Autodesk Inventor part; units mm, degrees
(part 6 of 6)
  line L4697 (26, 19.883) -> (26, 20.883)
  line L4698 (26, 20.883) -> (25, 20.883)
  line L4699 (25, 20.883) -> (25, 19.883)
  line L4700 (25, 20.383) -> (26, 20.383)
  line L4701 (26, 20.383) -> (26, 21.383)
  line L4702 (26, 21.383) -> (25, 21.383)
  line L4703 (25, 21.383) -> (25, 20.383)
  line L4704 (25, 20.883) -> (26, 20.883)
  line L4705 (26, 20.883) -> (26, 21.883)
  line L4706 (26, 21.883) -> (25, 21.883)
  line L4707 (25, 21.883) -> (25, 20.883)
  line L4708 (25, 21.383) -> (26, 21.383)
  line L4709 (26, 21.383) -> (26, 22.383)
  line L4710 (26, 22.383) -> (25, 22.383)
  line L4711 (25, 22.383) -> (25, 21.383)
  line L4712 (25, 21.883) -> (26, 21.883)
  line L4713 (26, 21.883) -> (26, 22.883)
  line L4714 (26, 22.883) -> (25, 22.883)
  line L4715 (25, 22.883) -> (25, 21.883)
  line L4716 (23.28, 23.603) -> (24.28, 23.603)
  line L4717 (24.28, 23.603) -> (24.28, 24.603)
  line L4718 (24.28, 24.603) -> (23.28, 24.603)
  line L4719 (23.28, 24.603) -> (23.28, 23.603)
  line L4720 (22.78, 23.603) -> (23.78, 23.603)
  line L4721 (23.78, 23.603) -> (23.78, 24.603)
  line L4722 (23.78, 24.603) -> (22.78, 24.603)
  line L4723 (22.78, 24.603) -> (22.78, 23.603)
  line L4724 (22.28, 23.603) -> (23.28, 23.603)
  line L4725 (23.28, 23.603) -> (23.28, 24.603)
  line L4726 (23.28, 24.603) -> (22.28, 24.603)
  line L4727 (22.28, 24.603) -> (22.28, 23.603)
  line L4728 (21.78, 23.603) -> (22.78, 23.603)
  line L4729 (22.78, 23.603) -> (22.78, 24.603)
  line L4730 (22.78, 24.603) -> (21.78, 24.603)
  line L4731 (21.78, 24.603) -> (21.78, 23.603)
  line L4732 (21.28, 23.603) -> (22.28, 23.603)
  line L4733 (22.28, 23.603) -> (22.28, 24.603)
  line L4734 (22.28, 24.603) -> (21.28, 24.603)
  line L4735 (21.28, 24.603) -> (21.28, 23.603)
  line L4736 (20.78, 23.603) -> (21.78, 23.603)
  line L4737 (21.78, 23.603) -> (21.78, 24.603)
  line L4738 (21.78, 24.603) -> (20.78, 24.603)
  line L4739 (20.78, 24.603) -> (20.78, 23.603)
  line L4740 (20.28, 23.603) -> (21.28, 23.603)
  line L4741 (21.28, 23.603) -> (21.28, 24.603)
  line L4742 (21.28, 24.603) -> (20.28, 24.603)
  line L4743 (20.28, 24.603) -> (20.28, 23.603)
  line L4744 (19.78, 23.603) -> (20.78, 23.603)
  line L4745 (20.78, 23.603) -> (20.78, 24.603)
  line L4746 (20.78, 24.603) -> (19.78, 24.603)
  line L4747 (19.78, 24.603) -> (19.78, 23.603)
  line L4748 (19.28, 23.603) -> (20.28, 23.603)
  line L4749 (20.28, 23.603) -> (20.28, 24.603)
  line L4750 (20.28, 24.603) -> (19.28, 24.603)
  line L4751 (19.28, 24.603) -> (19.28, 23.603)
  line L4752 (18.78, 23.603) -> (19.78, 23.603)
  line L4753 (19.78, 23.603) -> (19.78, 24.603)
  line L4754 (19.78, 24.603) -> (18.78, 24.603)
  line L4755 (18.78, 24.603) -> (18.78, 23.603)
  line L4756 (18.28, 23.603) -> (19.28, 23.603)
  line L4757 (19.28, 23.603) -> (19.28, 24.603)
  line L4758 (19.28, 24.603) -> (18.28, 24.603)
  line L4759 (18.28, 24.603) -> (18.28, 23.603)
  line L4760 (17.78, 23.603) -> (18.78, 23.603)
  line L4761 (18.78, 23.603) -> (18.78, 24.603)
  line L4762 (18.78, 24.603) -> (17.78, 24.603)
  line L4763 (17.78, 24.603) -> (17.78, 23.603)
  line L4764 (17.28, 23.603) -> (18.28, 23.603)
  line L4765 (18.28, 23.603) -> (18.28, 24.603)
  line L4766 (18.28, 24.603) -> (17.28, 24.603)
  line L4767 (17.28, 24.603) -> (17.28, 23.603)
  line L4768 (16.78, 23.603) -> (17.78, 23.603)
  line L4769 (17.78, 23.603) -> (17.78, 24.603)
  line L4770 (17.78, 24.603) -> (16.78, 24.603)
  line L4771 (16.78, 24.603) -> (16.78, 23.603)
  line L4772 (16.28, 23.603) -> (17.28, 23.603)
  line L4773 (17.28, 23.603) -> (17.28, 24.603)
  line L4774 (17.28, 24.603) -> (16.28, 24.603)
  line L4775 (16.28, 24.603) -> (16.28, 23.603)
  line L4776 (15.78, 23.603) -> (16.78, 23.603)
  line L4777 (16.78, 23.603) -> (16.78, 24.603)
  line L4778 (16.78, 24.603) -> (15.78, 24.603)
  line L4779 (15.78, 24.603) -> (15.78, 23.603)
  line L4780 (15.28, 23.603) -> (16.28, 23.603)
  line L4781 (16.28, 23.603) -> (16.28, 24.603)
  line L4782 (16.28, 24.603) -> (15.28, 24.603)
  line L4783 (15.28, 24.603) -> (15.28, 23.603)
  line L4784 (14.78, 23.603) -> (15.78, 23.603)
  line L4785 (15.78, 23.603) -> (15.78, 24.603)
  line L4786 (15.78, 24.603) -> (14.78, 24.603)
  line L4787 (14.78, 24.603) -> (14.78, 23.603)
  line L4788 (14.28, 23.603) -> (15.28, 23.603)
  line L4789 (15.28, 23.603) -> (15.28, 24.603)
  line L4790 (15.28, 24.603) -> (14.28, 24.603)
  line L4791 (14.28, 24.603) -> (14.28, 23.603)
  line L4792 (13.78, 23.603) -> (14.78, 23.603)
  line L4793 (14.78, 23.603) -> (14.78, 24.603)
  line L4794 (14.78, 24.603) -> (13.78, 24.603)
  line L4795 (13.78, 24.603) -> (13.78, 23.603)
  line L4796 (13.28, 23.603) -> (14.28, 23.603)
  line L4797 (14.28, 23.603) -> (14.28, 24.603)
  line L4798 (14.28, 24.603) -> (13.28, 24.603)
  line L4799 (13.28, 24.603) -> (13.28, 23.603)
  line L4800 (12.78, 23.603) -> (13.78, 23.603)
  line L4801 (13.78, 23.603) -> (13.78, 24.603)
  line L4802 (13.78, 24.603) -> (12.78, 24.603)
  line L4803 (12.78, 24.603) -> (12.78, 23.603)
  line L4804 (12.28, 23.603) -> (13.28, 23.603)
  line L4805 (13.28, 23.603) -> (13.28, 24.603)
  line L4806 (13.28, 24.603) -> (12.28, 24.603)
  line L4807 (12.28, 24.603) -> (12.28, 23.603)
  line L4808 (11.78, 23.603) -> (12.78, 23.603)
  line L4809 (12.78, 23.603) -> (12.78, 24.603)
  line L4810 (12.78, 24.603) -> (11.78, 24.603)
  line L4811 (11.78, 24.603) -> (11.78, 23.603)
  line L4812 (11.28, 23.603) -> (12.28, 23.603)
  line L4813 (12.28, 23.603) -> (12.28, 24.603)
  line L4814 (12.28, 24.603) -> (11.28, 24.603)
  line L4815 (11.28, 24.603) -> (11.28, 23.603)
  circle A74 centre (19.9, 34.55) radius 0.17
  circle A75 centre (19.1, 34.55) radius 0.17
  circle A76 centre (18.3, 34.55) radius 0.17
  circle A77 centre (17.5, 34.55) radius 0.17
  circle A78 centre (16.7, 34.55) radius 0.17
  circle A79 centre (15.9, 34.55) radius 0.17
  circle A80 centre (19.9, 35.3) radius 0.17
  circle A81 centre (19.1, 35.3) radius 0.17
  circle A82 centre (18.3, 35.3) radius 0.17
  circle A83 centre (17.5, 35.3) radius 0.17
  circle A84 centre (16.7, 35.3) radius 0.17
  circle A85 centre (15.9, 35.3) radius 0.17
  circle A86 centre (19.9, 36.05) radius 0.17
  circle A87 centre (15.9, 36.05) radius 0.17
  circle A88 centre (19.9, 36.8) radius 0.17
  circle A89 centre (15.9, 36.8) radius 0.17
  circle A90 centre (19.9, 37.55) radius 0.17
  circle A91 centre (19.1, 37.55) radius 0.17
  circle A92 centre (18.3, 37.55) radius 0.17
  circle A93 centre (17.5, 37.55) radius 0.17
  circle A94 centre (16.7, 37.55) radius 0.17
  circle A95 centre (15.9, 37.55) radius 0.17
  circle A96 centre (19.9, 38.3) radius 0.17
  circle A97 centre (19.1, 38.3) radius 0.17
  circle A98 centre (18.3, 38.3) radius 0.17
  circle A99 centre (17.5, 38.3) radius 0.17
  circle A100 centre (16.7, 38.3) radius 0.17
  circle A101 centre (15.9, 38.3) radius 0.17
  line L4816 (8.103, 5.199) -> (8.103, 4.199)
  line L4817 (8.103, 4.199) -> (9.103, 4.199)
  line L4818 (9.103, 4.199) -> (9.103, 5.199)
  line L4819 (9.103, 5.199) -> (8.103, 5.199)
  line L4820 (8.103, 3.929) -> (8.103, 2.929)
  line L4821 (8.103, 2.929) -> (9.103, 2.929)
  line L4822 (9.103, 2.929) -> (9.103, 3.929)
  line L4823 (9.103, 3.929) -> (8.103, 3.929)
  line L4824 (8.103, 2.659) -> (8.103, 1.659)
  line L4825 (8.103, 1.659) -> (9.103, 1.659)
  line L4826 (9.103, 1.659) -> (9.103, 2.659)
  line L4827 (9.103, 2.659) -> (8.103, 2.659)
  line L4828 (8.103, 1.389) -> (8.103, 0.389)
  line L4829 (8.103, 0.389) -> (9.103, 0.389)
  line L4830 (9.103, 0.389) -> (9.103, 1.389)
  line L4831 (9.103, 1.389) -> (8.103, 1.389)
  line L4832 (13.503, 1.389) -> (13.503, 0.389)
  line L4833 (13.503, 0.389) -> (14.503, 0.389)
  line L4834 (14.503, 0.389) -> (14.503, 1.389)
  line L4835 (14.503, 1.389) -> (13.503, 1.389)
  line L4836 (13.503, 2.659) -> (13.503, 1.659)
  line L4837 (13.503, 1.659) -> (14.503, 1.659)
  line L4838 (14.503, 1.659) -> (14.503, 2.659)
  line L4839 (14.503, 2.659) -> (13.503, 2.659)
  line L4840 (13.503, 3.929) -> (13.503, 2.929)
  line L4841 (13.503, 2.929) -> (14.503, 2.929)
  line L4842 (14.503, 2.929) -> (14.503, 3.929)
  line L4843 (14.503, 3.929) -> (13.503, 3.929)
  line L4844 (13.503, 5.199) -> (13.503, 4.199)
  line L4845 (13.503, 4.199) -> (14.503, 4.199)
  line L4846 (14.503, 4.199) -> (14.503, 5.199)
  line L4847 (14.503, 5.199) -> (13.503, 5.199)
  line L4848 (10.803, 3.294) -> (10.803, 2.294)
  line L4849 (10.803, 2.294) -> (11.803, 2.294)
  line L4850 (11.803, 2.294) -> (11.803, 3.294)
  line L4851 (11.803, 3.294) -> (10.803, 3.294)
  line L4852 (31.641, 22.218) -> (31.641, 21.068)
  line L4853 (31.641, 21.068) -> (32.791, 21.068)
  line L4854 (32.791, 21.068) -> (32.791, 22.218)
  line L4855 (32.791, 22.218) -> (31.641, 22.218)
  line L4856 (34.266, 22.143) -> (34.266, 21.143)
  line L4857 (34.266, 21.143) -> (35.266, 21.143)
  line L4858 (35.266, 21.143) -> (35.266, 22.143)
  line L4859 (35.266, 22.143) -> (34.266, 22.143)
  line L4860 (32.166, 32.593) -> (32.166, 31.593)
  line L4861 (32.166, 31.593) -> (33.166, 31.593)
  line L4862 (33.166, 31.593) -> (33.166, 32.593)
  line L4863 (33.166, 32.593) -> (32.166, 32.593)
  line L4864 (33.366, 32.793) -> (33.366, 31.793)
  line L4865 (33.366, 31.793) -> (34.366, 31.793)
  line L4866 (34.366, 31.793) -> (34.366, 32.793)
  line L4867 (34.366, 32.793) -> (33.366, 32.793)
  line L4868 (34.416, 32.593) -> (34.416, 31.593)
  line L4869 (34.416, 31.593) -> (35.416, 31.593)
  line L4870 (35.416, 31.593) -> (35.416, 32.593)
  line L4871 (35.416, 32.593) -> (34.416, 32.593)
  line L4872 (30.666, 30.943) -> (30.666, 29.943)
  line L4873 (30.666, 29.943) -> (31.666, 29.943)
  line L4874 (31.666, 29.943) -> (31.666, 30.943)
  line L4875 (31.666, 30.943) -> (30.666, 30.943)
  line L4876 (30.666, 29.843) -> (30.666, 28.843)
  line L4877 (30.666, 28.843) -> (31.666, 28.843)
  line L4878 (31.666, 28.843) -> (31.666, 29.843)
  line L4879 (31.666, 29.843) -> (30.666, 29.843)
  line L4880 (30.666, 28.743) -> (30.666, 27.743)
  line L4881 (30.666, 27.743) -> (31.666, 27.743)
  line L4882 (31.666, 27.743) -> (31.666, 28.743)
  line L4883 (31.666, 28.743) -> (30.666, 28.743)
  line L4884 (30.666, 27.643) -> (30.666, 26.643)
  line L4885 (30.666, 26.643) -> (31.666, 26.643)
  line L4886 (31.666, 26.643) -> (31.666, 27.643)
  line L4887 (31.666, 27.643) -> (30.666, 27.643)
  line L4888 (30.666, 26.543) -> (30.666, 25.543)
  line L4889 (30.666, 25.543) -> (31.666, 25.543)
  line L4890 (31.666, 25.543) -> (31.666, 26.543)
  line L4891 (31.666, 26.543) -> (30.666, 26.543)
  line L4892 (30.666, 25.443) -> (30.666, 24.443)
  line L4893 (30.666, 24.443) -> (31.666, 24.443)
  line L4894 (31.666, 24.443) -> (31.666, 25.443)
  line L4895 (31.666, 25.443) -> (30.666, 25.443)
  line L4896 (30.666, 24.343) -> (30.666, 23.343)
  line L4897 (30.666, 23.343) -> (31.666, 23.343)
  line L4898 (31.666, 23.343) -> (31.666, 24.343)
  line L4899 (31.666, 24.343) -> (30.666, 24.343)
  line L4900 (30.666, 23.243) -> (30.666, 22.243)
  line L4901 (30.666, 22.243) -> (31.666, 22.243)
  line L4902 (31.666, 22.243) -> (31.666, 23.243)
  line L4903 (31.666, 23.243) -> (30.666, 23.243)
  line L4904 (25.87, 4.6275) -> (24.87, 4.6275)
  line L4905 (24.87, 4.6275) -> (24.87, 3.6275)
  line L4906 (24.87, 3.6275) -> (25.87, 3.6275)
  line L4907 (25.87, 3.6275) -> (25.87, 4.6275)
  line L4908 (26.52, 4.6275) -> (25.52, 4.6275)
  line L4909 (25.52, 4.6275) -> (25.52, 3.6275)
  line L4910 (25.52, 3.6275) -> (26.52, 3.6275)
  line L4911 (26.52, 3.6275) -> (26.52, 4.6275)
  line L4912 (27.17, 4.6275) -> (26.17, 4.6275)
  line L4913 (26.17, 4.6275) -> (26.17, 3.6275)
  line L4914 (26.17, 3.6275) -> (27.17, 3.6275)
  line L4915 (27.17, 3.6275) -> (27.17, 4.6275)
  line L4916 (27.82, 4.6275) -> (26.82, 4.6275)
  line L4917 (26.82, 4.6275) -> (26.82, 3.6275)
  line L4918 (26.82, 3.6275) -> (27.82, 3.6275)
  line L4919 (27.82, 3.6275) -> (27.82, 4.6275)
  line L4920 (28.47, 4.6275) -> (27.47, 4.6275)
  line L4921 (27.47, 4.6275) -> (27.47, 3.6275)
  line L4922 (27.47, 3.6275) -> (28.47, 3.6275)
  line L4923 (28.47, 3.6275) -> (28.47, 4.6275)
  circle A102 centre (23.37, 1.4525) radius 0.935
  circle A103 centre (23.37, 1.4525) radius 0.935
  circle A104 centre (23.37, 1.4525) radius 0.935
  circle A105 centre (23.37, 1.4525) radius 0.935
  circle A106 centre (29.97, 1.4525) radius 0.935
  circle A107 centre (29.97, 1.4525) radius 0.935
  circle A108 centre (29.97, 1.4525) radius 0.935
  circle A109 centre (29.97, 1.4525) radius 0.935
  line L4924 (23.97, 3.6275) -> (23.97, 4.6275)
  line L4925 (23.97, 4.6275) -> (22.97, 4.6275)
  line L4926 (22.97, 4.6275) -> (22.97, 3.6275)
  line L4927 (22.97, 3.6275) -> (23.97, 3.6275)
  line L4928 (30.37, 3.6275) -> (30.37, 4.6275)
  line L4929 (30.37, 4.6275) -> (29.37, 4.6275)
  line L4930 (29.37, 4.6275) -> (29.37, 3.6275)
  line L4931 (29.37, 3.6275) -> (30.37, 3.6275)
  line L4932 (24.52, 0.5025) -> (26.42, 0.5025)
  line L4933 (26.42, 0.5025) -> (26.42, 2.4025)
  line L4934 (26.42, 2.4025) -> (24.52, 2.4025)
  line L4935 (24.52, 2.4025) -> (24.52, 0.5025)
  line L4936 (26.92, 0.5025) -> (28.82, 0.5025)
  line L4937 (28.82, 0.5025) -> (28.82, 2.4025)
  line L4938 (28.82, 2.4025) -> (26.92, 2.4025)
  line L4939 (26.92, 2.4025) -> (26.92, 0.5025)
  line L4940 (4.669, 18.214) -> (4.669, 17.214)
  line L4941 (4.669, 17.214) -> (5.669, 17.214)
  line L4942 (5.669, 17.214) -> (5.669, 18.214)
  line L4943 (5.669, 18.214) -> (4.669, 18.214)
  line L4944 (4.669, 16.364) -> (4.669, 15.364)
  line L4945 (4.669, 15.364) -> (5.669, 15.364)
  line L4946 (5.669, 15.364) -> (5.669, 16.364)
  line L4947 (5.669, 16.364) -> (4.669, 16.364)
  line L4948 (6.219, 16.364) -> (6.219, 15.364)
  line L4949 (6.219, 15.364) -> (7.219, 15.364)
  line L4950 (7.219, 15.364) -> (7.219, 16.364)
  line L4951 (7.219, 16.364) -> (6.219, 16.364)
  line L4952 (6.219, 18.214) -> (6.219, 17.214)
  line L4953 (6.219, 17.214) -> (7.219, 17.214)
  line L4954 (7.219, 17.214) -> (7.219, 18.214)
  line L4955 (7.219, 18.214) -> (6.219, 18.214)
  circle A110 centre (29.591, 23.622) radius 0.2286
  circle A111 centre (29.591, 23.622) radius 0.2286
  circle A112 centre (32.385, 14.224) radius 0.2286
  circle A113 centre (32.385, 14.224) radius 0.2286
  circle A114 centre (20.32, 18.034) radius 0.2286
  circle A115 centre (20.32, 18.034) radius 0.2286
  circle A116 centre (13.111, 7.6) radius 0.2286
  circle A117 centre (13.111, 7.6) radius 0.2286
  circle A118 centre (18.7, 37.15) radius 0.2286
  circle A119 centre (18.7, 37.15) radius 0.2286
  circle A120 centre (19.676, 22.67) radius 0.2286
  circle A121 centre (19.676, 22.67) radius 0.2286
  circle A122 centre (16.3, 38.7) radius 0.2286
  circle A123 centre (16.3, 38.7) radius 0.2286
  circle A124 centre (18.149, 21.651) radius 0.2286
  circle A125 centre (18.149, 21.651) radius 0.2286
  circle A126 centre (18.7, 38.7) radius 0.2286
  circle A127 centre (18.7, 38.7) radius 0.2286
  circle A128 centre (20.322, 20.778) radius 0.2286
  circle A129 centre (20.322, 20.778) radius 0.2286
  circle A130 centre (12.78, 35.731) radius 0.2286
  circle A131 centre (12.78, 35.731) radius 0.2286
  circle A132 centre (19.5, 37.15) radius 0.2286
  circle A133 centre (19.5, 37.15) radius 0.2286
  circle A134 centre (13, 22.3) radius 0.2286
  circle A135 centre (13, 22.3) radius 0.2286
  circle A136 centre (13.35, 35) radius 0.2286
  circle A137 centre (13.35, 35) radius 0.2286
  circle A138 centre (20.4, 37.15) radius 0.2286
  circle A139 centre (20.4, 37.15) radius 0.2286
  circle A140 centre (18.9, 28.573) radius 0.2286
  circle A141 centre (18.9, 28.573) radius 0.2286
  circle A142 centre (15.5, 38.7) radius 0.2286
  circle A143 centre (15.5, 38.7) radius 0.2286
  circle A144 centre (14.5, 22.3) radius 0.2286
  circle A145 centre (14.5, 22.3) radius 0.2286
  circle A146 centre (19.5, 38.7) radius 0.2286
  circle A147 centre (19.5, 38.7) radius 0.2286
  circle A148 centre (13.9, 20.7) radius 0.2286
  circle A149 centre (13.9, 20.7) radius 0.2286
  circle A150 centre (15.5, 34.925) radius 0.2286
  circle A151 centre (15.5, 34.925) radius 0.2286
  circle A152 centre (12.899, 9.58) radius 0.2286
  circle A153 centre (12.899, 9.58) radius 0.2286
  circle A154 centre (16.6, 36.65) radius 0.2286
  circle A155 centre (16.6, 36.65) radius 0.2286
  circle A156 centre (13.899, 9.58) radius 0.2286
  circle A157 centre (13.899, 9.58) radius 0.2286
  circle A158 centre (20.4, 36.4) radius 0.2286
  circle A159 centre (20.4, 36.4) radius 0.2286
  circle A160 centre (18.9, 27.273) radius 0.2286
  circle A161 centre (18.9, 27.273) radius 0.2286
  circle A162 centre (22.311, 22.097) radius 0.2286
  circle A163 centre (22.311, 22.097) radius 0.2286
  circle A164 centre (20.5, 33.1) radius 0.2286
  circle A165 centre (20.5, 33.1) radius 0.2286
  circle A166 centre (19.399, 26.384) radius 0.2286
  circle A167 centre (19.399, 26.384) radius 0.2286
  circle A168 centre (4.318, 20.701) radius 0.2286
  circle A169 centre (4.318, 20.701) radius 0.2286
  circle A170 centre (4.318, 16.764) radius 0.2286
  circle A171 centre (4.318, 16.764) radius 0.2286
  circle A172 centre (5.08, 12.827) radius 0.2286
  circle A173 centre (5.08, 12.827) radius 0.2286
  circle A174 centre (31.369, 32.512) radius 0.3658
  circle A175 centre (31.369, 32.512) radius 0.3658
  circle A176 centre (8.255, 21.717) radius 0.2972
  circle A177 centre (8.255, 21.717) radius 0.2972
  circle A178 centre (5.207, 20.701) radius 0.2286
  circle A179 centre (5.207, 20.701) radius 0.2286
  circle A180 centre (7.239, 12.827) radius 0.2286
  circle A181 centre (7.239, 12.827) radius 0.2286
  circle A182 centre (30.634, 18.515) radius 0.2972
  circle A183 centre (30.634, 18.515) radius 0.2972
  circle A184 centre (24.592, 22.079) radius 0.2972
  circle A185 centre (24.592, 22.079) radius 0.2972
  circle A186 centre (33.528, 21.717) radius 0.3657
  circle A187 centre (33.528, 21.717) radius 0.3657
  circle A188 centre (4.318, 18.161) radius 0.2286
  circle A189 centre (4.318, 18.161) radius 0.2286
  circle A190 centre (4.318, 15.113) radius 0.2286
  circle A191 centre (4.318, 15.113) radius 0.2286
  circle A192 centre (17.018, 0.635) radius 0.2972
  circle A193 centre (17.018, 0.635) radius 0.2972
  circle A194 centre (16.002, 0.635) radius 0.2972
  circle A195 centre (16.002, 0.635) radius 0.2972
  circle A196 centre (32.512, 24.638) radius 0.2972
  circle A197 centre (32.512, 24.638) radius 0.2972
  circle A198 centre (32.512, 25.4) radius 0.2972
  circle A199 centre (32.512, 25.4) radius 0.2972
  circle A200 centre (28.829, 5.461) radius 0.2972
  circle A201 centre (28.829, 5.461) radius 0.2972
  circle A202 centre (27.94, 5.461) radius 0.2972
  circle A203 centre (27.94, 5.461) radius 0.2972
  circle A204 centre (16.002, 1.397) radius 0.2972
  circle A205 centre (16.002, 1.397) radius 0.2972
  circle A206 centre (17.018, 1.397) radius 0.2972
  circle A207 centre (17.018, 1.397) radius 0.2972
  circle A208 centre (4.699, 0.635) radius 0.2972
  circle A209 centre (4.699, 0.635) radius 0.2972
  circle A210 centre (4.699, 1.524) radius 0.2972
  circle A211 centre (4.699, 1.524) radius 0.2972
  circle A212 centre (4.699, 2.413) radius 0.2972
  circle A213 centre (4.699, 2.413) radius 0.2972
  circle A214 centre (6.223, 12.827) radius 0.2286
  circle A215 centre (6.223, 12.827) radius 0.2286
  circle A216 centre (7.239, 20.701) radius 0.2286
  circle A217 centre (7.239, 20.701) radius 0.2286
  circle A218 centre (11.303, 17.653) radius 0.2972
  circle A219 centre (11.303, 17.653) radius 0.2972
  circle A220 centre (6.223, 20.701) radius 0.2286
  circle A221 centre (6.223, 20.701) radius 0.2286
  circle A222 centre (11.176, 26.289) radius 0.2972
  circle A223 centre (11.176, 26.289) radius 0.2972
  circle A224 centre (12.065, 26.289) radius 0.2972
  circle A225 centre (12.065, 26.289) radius 0.2972
  circle A226 centre (6.604, 8.509) radius 0.3048
  circle A227 centre (6.604, 8.509) radius 0.3048
  circle A228 centre (8.255, 8.509) radius 0.3048
  circle A229 centre (8.255, 8.509) radius 0.3048
  circle A230 centre (10.287, 6.477) radius 0.3048
  circle A231 centre (10.287, 6.477) radius 0.3048
  circle A232 centre (17.907, 6.477) radius 0.3048
  circle A233 centre (17.907, 6.477) radius 0.3048
  circle A234 centre (1.143, 27.051) radius 0.3657
  circle A235 centre (1.143, 27.051) radius 0.3657
  circle A236 centre (4.4958, 22.987) radius 0.3657
  circle A237 centre (4.4958, 22.987) radius 0.3657
  circle A238 centre (25.527, 26.797) radius 0.3048
  circle A239 centre (25.527, 26.797) radius 0.3048
  circle A240 centre (25.527, 5.969) radius 0.3048
  circle A241 centre (25.527, 5.969) radius 0.3048
  circle A242 centre (32.512, 26.162) radius 0.2972
  circle A243 centre (32.512, 26.162) radius 0.2972
  circle A244 centre (12.192, 4.064) radius 0.2972
  circle A245 centre (12.192, 4.064) radius 0.2972
  circle A246 centre (12.192, 1.524) radius 0.2972
  circle A247 centre (12.192, 1.524) radius 0.2972
  circle A248 centre (10.414, 1.524) radius 0.2972
  circle A249 centre (10.414, 1.524) radius 0.2972
  circle A250 centre (10.414, 4.064) radius 0.2972
  circle A251 centre (10.414, 4.064) radius 0.2972
  circle A252 centre (11.303, 4.064) radius 0.2972
  circle A253 centre (11.303, 4.064) radius 0.2972
  circle A254 centre (11.303, 1.524) radius 0.2972
  circle A255 centre (11.303, 1.524) radius 0.2972
  circle A256 centre (16.873, 41.6) radius 0.2972
  circle A257 centre (16.873, 41.6) radius 0.2972
  circle A258 centre (23, 35.1) radius 0.2972
  circle A259 centre (23, 35.1) radius 0.2972
  circle A260 centre (22.127, 30.273) radius 0.3657
  circle A261 centre (22.127, 30.273) radius 0.3657
  circle A262 centre (18.8, 31.0635) radius 0.2972
  circle A263 centre (18.8, 31.0635) radius 0.2972
  circle A264 centre (11.303, 13.208) radius 0.2972
  circle A265 centre (11.303, 13.208) radius 0.2972
  circle A266 centre (26.5746, 23.641) radius 0.2286
  circle A267 centre (26.5746, 23.641) radius 0.2286
  circle A268 centre (21.209, 30.099) radius 0.2972
  circle A269 centre (21.209, 30.099) radius 0.2972
  circle A270 centre (11.176, 25.527) radius 0.2972
  circle A271 centre (11.176, 25.527) radius 0.2972
  circle A272 centre (24.638, 40.767) radius 0.3657
  circle A273 centre (24.638, 40.767) radius 0.3657
  circle A274 centre (11.811, 35.687) radius 0.3657
  circle A275 centre (11.811, 35.687) radius 0.3657
  circle A276 centre (21.59, 9.779) radius 0.2286
  circle A277 centre (21.59, 9.779) radius 0.2286
  circle A278 centre (22.479, 9.779) radius 0.2286
  circle A279 centre (22.479, 9.779) radius 0.2286
  circle A280 centre (11.303, 14.097) radius 0.2286
  circle A281 centre (11.303, 14.097) radius 0.2286
  circle A282 centre (8.071, 29.953) radius 0.2286
  circle A283 centre (8.071, 29.953) radius 0.2286
  circle A284 centre (11.303, 14.883) radius 0.2286
  circle A285 centre (11.303, 14.883) radius 0.2286
  circle A286 centre (8.071, 30.753) radius 0.2286
  circle A287 centre (8.071, 30.753) radius 0.2286
  circle A288 centre (11.303, 15.621) radius 0.2286
  circle A289 centre (11.303, 15.621) radius 0.2286
  circle A290 centre (8.071, 31.553) radius 0.2286
  circle A291 centre (8.071, 31.553) radius 0.2286
  circle A292 centre (23, 36.7) radius 0.2972
  circle A293 centre (23, 36.7) radius 0.2972
  circle A294 centre (3.556, 25.019) radius 0.3657
  circle A295 centre (3.556, 25.019) radius 0.3657
  circle A296 centre (2.413, 33.528) radius 0.3657
  circle A297 centre (2.413, 33.528) radius 0.3657
  circle A298 centre (20.32, 16.256) radius 0.2286
  circle A299 centre (20.32, 16.256) radius 0.2286
  circle A300 centre (29.591, 24.384) radius 0.2286
  circle A301 centre (29.591, 24.384) radius 0.2286
  circle A302 centre (19.304, 0.635) radius 0.2972
  circle A303 centre (19.304, 0.635) radius 0.2972
  circle A304 centre (19.304, 1.397) radius 0.2972
  circle A305 centre (19.304, 1.397) radius 0.2972
  circle A306 centre (18.161, 1.397) radius 0.2972
  circle A307 centre (18.161, 1.397) radius 0.2972
  circle A308 centre (18.161, 0.635) radius 0.2972
  circle A309 centre (18.161, 0.635) radius 0.2972
  circle A310 centre (30.226, 26.035) radius 0.2286
  circle A311 centre (30.226, 26.035) radius 0.2286
  circle A312 centre (21.117, 26.019) radius 0.2286
  circle A313 centre (21.117, 26.019) radius 0.2286
  circle A314 centre (29.591, 22.86) radius 0.2286
  circle A315 centre (29.591, 22.86) radius 0.2286
  circle A316 centre (26.416, 17.272) radius 0.2286
  circle A317 centre (26.416, 17.272) radius 0.2286
  circle A318 centre (29.591, 22.098) radius 0.2286
  circle A319 centre (29.591, 22.098) radius 0.2286
  circle A320 centre (26.416, 18.034) radius 0.2286
  circle A321 centre (26.416, 18.034) radius 0.2286
  circle A322 centre (22.7838, 26.035) radius 0.2286
  circle A323 centre (22.7838, 26.035) radius 0.2286
  circle A324 centre (29.591, 31.115) radius 0.2286
  circle A325 centre (29.591, 31.115) radius 0.2286
  circle A326 centre (21.971, 26.035) radius 0.2286
  circle A327 centre (21.971, 26.035) radius 0.2286
  circle A328 centre (29.591, 30.353) radius 0.2286
  circle A329 centre (29.591, 30.353) radius 0.2286
  circle A330 centre (29.591, 31.9278) radius 0.2286
  circle A331 centre (29.591, 31.9278) radius 0.2286
  circle A332 centre (23.622, 26.035) radius 0.2286
  circle A333 centre (23.622, 26.035) radius 0.2286
  circle A334 centre (11.303, 11.176) radius 0.2286
  circle A335 centre (11.303, 11.176) radius 0.2286
  circle A336 centre (11.303, 12.065) radius 0.2286
  circle A337 centre (11.303, 12.065) radius 0.2286
  circle A338 centre (23.78, 22.956) radius 0.2286
  circle A339 centre (23.78, 22.956) radius 0.2286
  circle A340 centre (23.876, 13.208) radius 0.2286
  circle A341 centre (23.876, 13.208) radius 0.2286
  circle A342 centre (23.876, 13.97) radius 0.2286
  circle A343 centre (23.876, 13.97) radius 0.2286
  circle A344 centre (28.956, 10.922) radius 0.2286
  circle A345 centre (28.956, 10.922) radius 0.2286
  circle A346 centre (23.876, 14.732) radius 0.2286
  circle A347 centre (23.876, 14.732) radius 0.2286
  circle A348 centre (22.098, 5.461) radius 0.2972
  circle A349 centre (22.098, 5.461) radius 0.2972
  circle A350 centre (26.797, 8.382) radius 0.2972
  circle A351 centre (26.797, 8.382) radius 0.2972
  circle A352 centre (11.303, 19.558) radius 0.2972
  circle A353 centre (11.303, 19.558) radius 0.2972
  circle A354 centre (25.527, 23.114) radius 0.2972
  circle A355 centre (25.527, 23.114) radius 0.2972
  circle A356 centre (32.512, 27.178) radius 0.2972
  circle A357 centre (32.512, 27.178) radius 0.2972
  circle A358 centre (32.512, 28.194) radius 0.2972
  circle A359 centre (32.512, 28.194) radius 0.2972
  circle A360 centre (5.715, 6.477) radius 0.2972
  circle A361 centre (5.715, 6.477) radius 0.2972
  circle A362 centre (4.699, 6.477) radius 0.2972
  circle A363 centre (4.699, 6.477) radius 0.2972
  circle A364 centre (6.731, 6.477) radius 0.2972
  circle A365 centre (6.731, 6.477) radius 0.2972
  circle A366 centre (11.176, 24.511) radius 0.2972
  circle A367 centre (11.176, 24.511) radius 0.2972
  circle A368 centre (8.255, 17.907) radius 0.2972
  circle A369 centre (8.255, 17.907) radius 0.2972
  circle A370 centre (4.318, 32.766) radius 0.2972
  circle A371 centre (4.318, 32.766) radius 0.2972
  circle A372 centre (11.176, 23.711) radius 0.2972
  circle A373 centre (11.176, 23.711) radius 0.2972
  circle A374 centre (6.731, 5.588) radius 0.2972
  circle A375 centre (6.731, 5.588) radius 0.2972
  circle A376 centre (5.715, 5.588) radius 0.2972
  circle A377 centre (5.715, 5.588) radius 0.2972
  circle A378 centre (4.953, 8.509) radius 0.3048
  circle A379 centre (4.953, 8.509) radius 0.3048
  circle A380 centre (13.843, 6.477) radius 0.3048
  circle A381 centre (13.843, 6.477) radius 0.3048
  circle A382 centre (25.527, 9.652) radius 0.3048
  circle A383 centre (25.527, 9.652) radius 0.3048
  circle A384 centre (4.699, 3.429) radius 0.2972
  circle A385 centre (4.699, 3.429) radius 0.2972
  circle A386 centre (4.699, 4.445) radius 0.2972
  circle A387 centre (4.699, 4.445) radius 0.2972
  circle A388 centre (4.699, 5.588) radius 0.2972
  circle A389 centre (4.699, 5.588) radius 0.2972
  circle A390 centre (3.302, 32.766) radius 0.2972
  circle A391 centre (3.302, 32.766) radius 0.2972
  circle A392 centre (15, 33.1) radius 0.2286
  circle A393 centre (15, 33.1) radius 0.2286
  circle A394 centre (26.5746, 22.041) radius 0.2286
  circle A395 centre (26.5746, 22.041) radius 0.2286
  circle A396 centre (26.5746, 22.841) radius 0.2286
  circle A397 centre (26.5746, 22.841) radius 0.2286
  circle A398 centre (26.5746, 24.441) radius 0.2286
  circle A399 centre (26.5746, 24.441) radius 0.2286
  circle A400 centre (26.524, 31.934) radius 0.2286
  circle A401 centre (26.524, 31.934) radius 0.2286
  circle A402 centre (26.524, 31.134) radius 0.2286
  circle A403 centre (26.524, 31.134) radius 0.2286
  circle A404 centre (26.524, 30.334) radius 0.2286
  circle A405 centre (26.524, 30.334) radius 0.2286
  circle A406 centre (26.524, 29.534) radius 0.2286
  circle A407 centre (26.524, 29.534) radius 0.2286
  circle A408 centre (33.274, 33.655) radius 0.3657
  circle A409 centre (33.274, 33.655) radius 0.3657
  circle A410 centre (23.7, 30.304) radius 0.3657
  circle A411 centre (23.7, 30.304) radius 0.3657
  circle A412 centre (21.971, 40.767) radius 0.3657
  circle A413 centre (21.971, 40.767) radius 0.3657
  circle A414 centre (8.128, 25.273) radius 0.3657
  circle A415 centre (8.128, 25.273) radius 0.3657
  circle A416 centre (12.065, 39.497) radius 0.3657
  circle A417 centre (12.065, 39.497) radius 0.3657
  constraints: 9912 end point, 418 centre point, 6 point on circle
chamfer "面取り2" distance 2 angle 45 2 edges at (38.06, -1.8075, 0) (6.39, -1.8075, 0)
chamfer "面取り3" distance 0.5 angle 45 2 edges at (6.39, -3.6273, 5) (38.06, -3.6273, 5)
